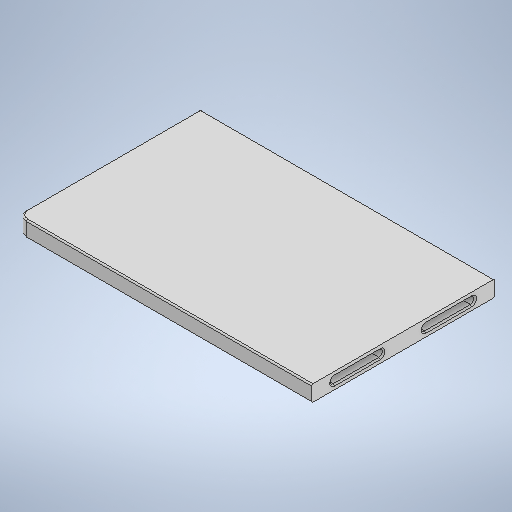
# Autodesk Inventor part: LeftClamo3
Saved by Autodesk Inventor 2025.3 (Build 293356000, 356)
## iProperties
Created: 2025-11-20
Part Number: LeftClamo3
Material: Generic
Document SubType Name: Modeling
Designer: User
Density: 1 g/cm^3
Appearance: Default
Author: User
Autodesk Inventor part; units mm, degrees
ref_plane "YZ Plane" through (0, 0, 0) normal (1, 0, 0) x (0, 1, 0)
ref_plane "XZ Plane" through (0, 0, 0) normal (0, 1, 0) x (-1, 0, 0)
sketch "Sketch1" plane through (0, 0, 0) normal (0, 1, 0) x (-1, 0, 0)
  line L0 (0, 0) -> (420, 0)
  line L1 (420, 0) -> (420, -40)
  line L2 (420, -40) -> (0, -40)
  line L3 (0, -40) -> (0, 0)
  dimension "d0" = 420
  dimension "d1" = 40
  constraints: 8 end point, 2 parallel, 1 horizontal, 1 perpendicular
  measures "d0" distance of L1.end L2.end
  measures "d1" distance of L0.end L1.end
extrude "Extrusion1" add sketch "Sketch1" along normal blind 3.5
fillet "Fillet1" radius 0.3 10 edges at (-210, 3.5, 0) (-210, 0, 0) (0, 0, -20) (0, 3.5, -20) (0, 1.75, -40) (-210, 3.5, -40) (-210, 0, -40) (-420, 0, -20) (-420, 1.75, -40) (-420, 3.5, -20)
sketch "Sketch2" plane through (0, 0, 0) normal (0, -1, 0) x (1, 0, 0)
  line L0 (-419.7, -39.7) -> (-419.7, -0.3) projected
  line L1 (-419.7, -20) -> (0, -20)
  circle A0 centre (-405, -20) radius 5
  circle A1 centre (-375, -20) radius 5
  circle A2 centre (-345, -20) radius 5
  circle A3 centre (-315, -20) radius 5
  line L2 (-420, 0) -> (-420, -39.7) projected
  line L3 (-315, -20) -> (-315, -8.0411)
  line L4 (-210.3, -20) -> (-630, -20)
  circle A4 centre (-225, -20) radius 5
  circle A5 centre (-255, -20) radius 5
  circle A6 centre (-285, -20) radius 5
  point P0 (0, 0)
  point P1 (-420, -0.3)
  dimension "d5" = 10
  dimension "d6" = 10
  dimension "d7" = 10
  dimension "d8" = 10
  dimension "d9" = 15
  dimension "d10" = 30
  dimension "d11" = 30
  dimension "d12" = 30
  constraints: 7 centre point, 7 point on line, 6 end point, 5 symmetric about line, 1 horizontal, 1 midpoint, 1 vertical, 3 other
  measures "d5" diameter of A0
  measures "d6" diameter of A1
  measures "d7" diameter of A2
  measures "d8" diameter of A3
  measures "d9" distance from line of L2 A0.centre
  measures "d10" distance of A1.centre A0.centre
  measures "d11" distance of A2.centre A1.centre
  measures "d12" distance of L3.start A2.centre
ref_plane "Work Plane1" through (-210, 0.3, -39.7) normal (1, 0, 0) x (0, 0, -1)
extrude "Extrusion2" cut sketch "Sketch2" against normal blind 3
mirror "Mirror1" about plane through (-210, 0.3, -39.7) normal (1, 0, 0) of "Extrusion2"
fillet "Fillet2" radius 2 6 edges at (-0.0879, 3.4121, -0.0879) (-0.0879, 0.0879, -0.0879) (0, 1.75, 0) (-419.9121, 3.4121, -0.0879) (-419.9121, 0.0879, -0.0879) (-420, 1.75, 0)
sketch "Sketch3" plane through (0, 3.5, 0) normal (0, 1, 0) x (1, 0, 0)
  line L0 (4.2695, -58.2258) -> (-175.7305, -58.2258)
  line L1 (-175.7305, -58.2258) -> (-175.7305, 85.9661)
  line L2 (-175.7305, 85.9661) -> (4.2695, 85.9661)
  line L3 (4.2695, 85.9661) -> (4.2695, -58.2258)
  line L4 (-175.7305, 85.9661) -> (-355.7305, 85.9661)
  line L5 (-355.7305, 85.9661) -> (-355.7305, -58.2258)
  line L6 (-355.7305, -58.2258) -> (-175.7305, -58.2258)
  line L7 (-175.7305, -58.2258) -> (-175.7305, 85.9661)
  line L8 (-355.7305, -58.2258) -> (-453.8172, -58.2258)
  line L9 (-453.8172, -58.2258) -> (-453.8172, 85.9661)
  line L10 (-453.8172, 85.9661) -> (-355.7305, 85.9661)
  line L11 (-355.7305, 85.9661) -> (-355.7305, -58.2258)
  point P0 (0, 0)
  dimension "d18" = 180
  dimension "d19" = 180
  constraints: 24 end point, 6 parallel, 3 horizontal, 3 perpendicular, 1 point on line
  measures "d18" distance of L1.end L2.end
  measures "d19" distance of L6.end L5.end
extrude "Extrusion8" cut sketch "Sketch3" against normal through all contours L0 L1 L2 L3 | L6 L5 L4 L1
sketch "Sketch7" plane through (-355.7305, 3.5, -0.3) normal (1, 0, 0) x (0, 0, -1)
  line L0 (4.7, -1.75) -> (14.7, -1.75) construction
  line L1 (-0.3, -3.2) -> (-0.3, -0.3) projected
  line L2 (4.7, -2.5) -> (14.7, -2.5)
  line L3 (14.7, -1) -> (4.7, -1)
  arc A0 (4.7, -1) -> (4.7, -2.5) centre (4.7, -1.75) ccw
  arc A1 (14.7, -2.5) -> (14.7, -1) centre (14.7, -1.75) ccw
  line L4 (24.7, -1.75) -> (34.7, -1.75) construction
  line L5 (24.7, -2.5) -> (34.7, -2.5)
  line L6 (34.7, -1) -> (24.7, -1)
  arc A2 (24.7, -1) -> (24.7, -2.5) centre (24.7, -1.75) ccw
  arc A3 (34.7, -2.5) -> (34.7, -1) centre (34.7, -1.75) ccw
  line L7 (39.7, -0.3) -> (39.7, -3.2) projected
  point P0 (-0.3, -3.5)
  point P1 (9.7, -1.75)
  point P2 (29.7, -1.75)
  dimension "d56" = 5
  dimension "d57" = 1.5
  dimension "d58" = 5
  dimension "d59" = 1.5
  dimension "d60" = 10
  dimension "d61" = 10
  constraints: 16 end point, 8 point on circle, 8 tangent, 4 centre point, 2 midpoint, 2 parallel, 2 point on line, 1 perpendicular
  measures "d56" distance of point (9.7, -1.75) L0.end
  measures "d57" diameter of A1
  measures "d58" distance of point (29.7, -1.75) L4.end
  measures "d59" diameter of A3
  measures "d60" distance from line of L7 point (29.7, -1.75)
  measures "d61" distance from line of L1 point (9.7, -1.75)
extrude "Extrusion9" cut sketch "Sketch7" against normal blind 16
chamfer "Chamfer3" distance 0.3 angle 45 8 edges at (-355.7305, 2.5, -10) (-355.7305, 1.75, -15.75) (-355.7305, 1, -10) (-355.7305, 1.75, -4.25) (-355.7305, 1.75, -24.25) (-355.7305, 2.5, -30) (-355.7305, 1.75, -35.75) (-355.7305, 1, -30)
body "Solid1"
